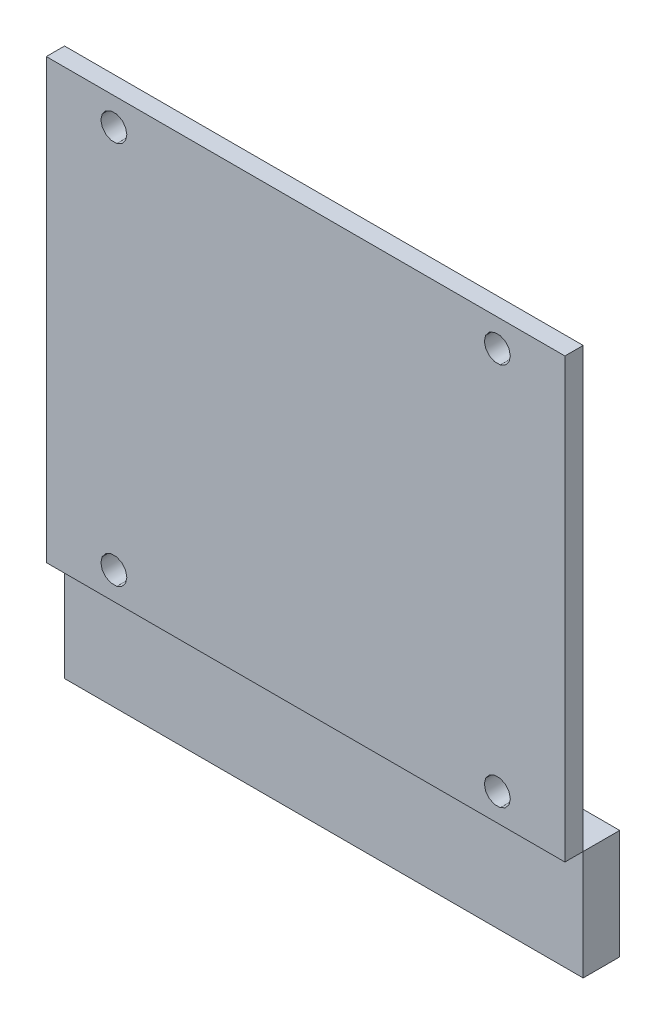
# Autodesk Inventor part: Fan_Mount
Saved by Autodesk Inventor 2023 (Build 270158000, 158)
## iProperties
Created: 2023-08-19
Part Number: Fan_Mount
Material: Generic
Document SubType Name: Modeling
Designer: plebbb
Density: 1 g/cm^3
Appearance: Default
Author: plebbb
Autodesk Inventor part; units mm, degrees
ref_plane "YZ Plane" through (0, 0, 0) normal (1, 0, 0) x (0, 1, 0)
ref_plane "XZ Plane" through (0, 0, 0) normal (0, 1, 0) x (-1, 0, 0)
ref_plane "XY Plane" through (0, 0, 0) normal (0, 0, 1) x (1, 0, 0)
sketch "Sketch1" plane through (0, 0, 0) normal (0, 0, 1) x (1, 0, 0)
  line L0 (0, 0) -> (142, 0)
  line L1 (142, 0) -> (142, 30)
  line L2 (142, 30) -> (0, 30)
  line L3 (0, 30) -> (0, 0)
  dimension "d0" = 30
  dimension "d1" = 142
  constraints: 8 end point, 2 parallel, 1 horizontal, 1 perpendicular
  measures "d0" distance of L0.end L1.end
  measures "d1" distance of L1.end L2.end
extrude "Extrusion1" add sketch "Sketch1" along normal blind 10
sketch "Sketch2" plane through (0, 0, 10) normal (0, 0, 1) x (1, 0, 0)
  line L0 (0, 30) -> (0, 0) projected
  line L1 (0, 30) -> (142, 30)
  line L2 (142, 30) -> (142, 150)
  line L3 (142, 150) -> (0, 150)
  line L4 (0, 150) -> (0, 30)
  dimension "d4" = 120
  constraints: 8 end point, 2 parallel, 1 coincident, 1 horizontal, 1 perpendicular
  measures "d4" distance of L1.end L2.end
extrude "Extrusion2" add sketch "Sketch2" along normal blind 5
sketch "Sketch3" plane through (0, 0, 15) normal (0, 0, 1) x (1, 0, 0)
  line L0 (142, 30) -> (142, 150) construction
  line L1 (142, 150) -> (0, 150) construction
  line L2 (0, 150) -> (0, 30) construction
  line L3 (0, 30) -> (142, 30) construction
  line L4 (18.5, 142.5) -> (123.5, 142.5) construction
  line L5 (123.5, 142.5) -> (123.5, 37.5) construction
  line L6 (123.5, 37.5) -> (18.5, 37.5) construction
  line L7 (18.5, 37.5) -> (18.5, 142.5) construction
  line L8 (142, 150) -> (0, 150) projected
  line L9 (71, 150) -> (71, 142.5) construction
  circle A0 centre (18.5, 142.5) radius 3.556
  circle A1 centre (123.5, 142.5) radius 3.556
  circle A2 centre (123.5, 37.5) radius 3.556
  circle A3 centre (18.5, 37.5) radius 3.556
  line L10 (71, 37.5) -> (71, 30) construction
  point P0 (0, 0)
  dimension "d7" = 105
  dimension "d8" = 7.112
  constraints: 12 end point, 4 centre point, 4 coincident, 4 equal length, 4 midpoint, 3 equal radius, 2 parallel, 1 horizontal, 1 perpendicular, 1 vertical
  measures "d7" distance of L4.start L4.end
  measures "d8" diameter of A0
extrude "Extrusion3" cut sketch "Sketch3" against normal blind 5
body "Solid1"
